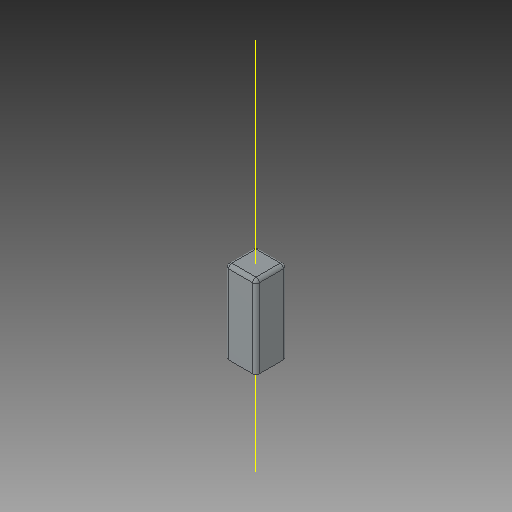
# Autodesk Inventor part: One_sided_axle_base-02-01
Saved by Autodesk Inventor 2019.3 (Build 233278000, 278)
## iProperties
Company: Unknown
Created: 2018-11-05
Part Number: One_sided_axle_base-02-01
Material: Generic
Description: Unknown
Document SubType Name: Modeling
Designer: Varga Daniel
Density: 1 g/cm^3
Appearance: Default
Sending System: DEX
Preprocessor: ST-DEVELOPER v16.7
Axle_length: 10,000 mm
Upper_fillet: 0,400 mm
Title: Axeis 2
Author: Unknown
Autodesk Inventor part; units mm, degrees
ref_plane "YZ Plane" through (0, 0, 0) normal (1, 0, 0) x (0, 1, 0)
ref_plane "XZ Plane" through (0, 0, 0) normal (0, 1, 0) x (-1, 0, 0)
ref_plane "XY Plane" through (0, 0, 0) normal (0, 0, 1) x (1, 0, 0)
derived "Base_part.ipt"
sketch "Axle_sketch" plane through (0, 0, 0) normal (0, 1, 0) x (-1, 0, 0)
  circle A0 centre (-15.8957, 4.3197) radius 2.5 construction
  line L0 (-14.4207, 2.4447) -> (-17.3707, 2.4447)
  line L1 (-17.7707, 2.8447) -> (-17.7707, 5.7947)
  line L2 (-17.3707, 6.1947) -> (-14.4207, 6.1947)
  line L3 (-14.0207, 5.7947) -> (-14.0207, 2.8447)
  line L4 (-14.0207, 2.4447) -> (-17.7707, 6.1947) construction
  line L5 (-17.7707, 2.4447) -> (-14.0207, 6.1947) construction
  arc A1 (-14.4207, 2.4447) -> (-14.0207, 2.8447) centre (-14.4207, 2.8447) ccw
  arc A2 (-17.7707, 2.8447) -> (-17.3707, 2.4447) centre (-17.3707, 2.8447) ccw
  arc A3 (-14.0207, 5.7947) -> (-14.4207, 6.1947) centre (-14.4207, 5.7947) ccw
  arc A4 (-17.3707, 6.1947) -> (-17.7707, 5.7947) centre (-17.3707, 5.7947) ccw
  point P0 (0, 0)
sketch "Sketch1" plane through (0, 0, 0) normal (0, 1, 0) x (-1, 0, 0)
  line L0 (-1.475, -1.875) -> (1.475, -1.875)
  line L1 (1.875, -1.475) -> (1.875, 1.475)
  line L2 (1.475, 1.875) -> (-1.475, 1.875)
  line L3 (-1.875, 1.475) -> (-1.875, -1.475)
  line L4 (-1.875, -1.875) -> (1.875, 1.875) construction
  line L5 (1.875, -1.875) -> (-1.875, 1.875) construction
  arc A0 (-1.875, -1.475) -> (-1.475, -1.875) centre (-1.475, -1.475) ccw
  arc A1 (1.475, -1.875) -> (1.875, -1.475) centre (1.475, -1.475) ccw
  arc A2 (1.875, 1.475) -> (1.475, 1.875) centre (1.475, 1.475) ccw
  arc A3 (-1.475, 1.875) -> (-1.875, 1.475) centre (-1.475, 1.475) ccw
  circle A4 centre (0, 0) radius 2.5 construction
  line L6 (-14.4207, 2.4447) -> (-17.3707, 2.4447) construction
  arc A5 (-14.4207, 2.4447) -> (-14.0207, 2.8447) centre (-14.4207, 2.8447) ccw construction
  line L7 (-14.0207, 5.7947) -> (-14.0207, 2.8447) construction
  circle A6 centre (-15.8957, 4.3197) radius 2.5 construction
  line L8 (-17.3707, 6.1947) -> (-14.4207, 6.1947) construction
  arc A7 (-17.3707, 6.1947) -> (-17.7707, 5.7947) centre (-17.3707, 5.7947) ccw construction
  line L9 (-17.7707, 2.8447) -> (-17.7707, 5.7947) construction
  arc A8 (-17.7707, 2.8447) -> (-17.3707, 2.4447) centre (-17.3707, 2.8447) ccw construction
  arc A9 (-14.0207, 5.7947) -> (-14.4207, 6.1947) centre (-14.4207, 5.7947) ccw construction
  dimension "d0" = 3.75
  dimension "d1" = 3.75
  dimension "d2" = 0.4
  dimension "d11" = 5
  dimension "d13" = 3.75
  dimension "d14" = 0.4
  constraints: 12 end point, 8 point on circle, 8 point on line, 8 tangent, 5 centre point, 3 equal radius, 2 midpoint, 2 parallel, 1 coincident, 1 horizontal, 1 perpendicular
  measures "d0" distance of L4.end L5.end
  measures "d1" distance between parallel lines of L2 L0
  measures "d2" radius of A0
  measures "d11" diameter of A4
  measures "d13" distance between parallel lines of L7 L9
  measures "d14" radius of A8
extrude "Extrusion4" add sketch "Sketch1" along normal blind 10
fillet "Fillet2" radius 0.4 8 edges at (1.7578, 10, -1.7578) (0, 10, -1.875) (-1.7578, 10, -1.7578) (-1.875, 10, 0) (-1.7578, 10, 1.7578) (0, 10, 1.875) (1.7578, 10, 1.7578) (1.875, 10, 0)
ref_plane "Work Plane3" through (-1.475, 0, 0) normal (0, 0, 1) x (1, 0, 0)
ref_plane "Work Plane4" through (0, 0, -1.475) normal (-1, 0, 0) x (0, 0, 1)
equation "\"d0\" = d13"
equation "\"d1\" = d0"
equation "\"d2\" = d14"
equation "\"d15\" = Axle_length"
equation "\"d17\" = Upper_fillet"
equation "\"Axle_length\" = 10"
equation "\"Upper_fillet\" = Axle_fillet"
equation "\"Axle_fillet\" = 0.4"
body "Solid1"
